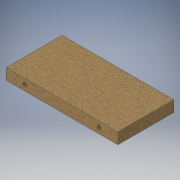
# Autodesk Inventor part: AkkuHaltSeitenWand
Saved by Autodesk Inventor 2017 SP1 (Build 210196100, 196)
## iProperties
Part Number: AkkuHaltSeitenWand
Material: Generisch
Document SubType Name: Modeling
Designer: Alex
Density: 1 g/cm^3
Appearance: Vorgabe
Author: Alex
Autodesk Inventor part; units mm, degrees
ref_plane "YZ Plane" through (0, 0, 0) normal (1, 0, 0) x (0, 1, 0)
ref_plane "XZ Plane" through (0, 0, 0) normal (0, 1, 0) x (-1, 0, 0)
ref_plane "XY Plane" through (0, 0, 0) normal (0, 0, 1) x (1, 0, 0)
sketch "Skizze1" plane through (0, 0, 0) normal (0, 1, 0) x (-1, 0, 0)
  line L0 (0, 0) -> (60, 0)
  line L1 (60, 0) -> (60, -6)
  line L2 (60, -6) -> (0, -6)
  line L3 (0, -6) -> (0, 0)
  dimension "d0" = 60
  dimension "d1" = 6
  constraints: 8 end point, 2 parallel, 1 horizontal, 1 perpendicular
  measures "d0" distance of L1.end L2.end
  measures "d1" distance of L0.end L1.end
extrude "Extrusion1" add sketch "Skizze1" along normal blind 30
sketch "m" plane through (0, 0, 0) normal (0, -1, 0) x (1, 0, 0)
  line L0 (0, -6) -> (0, 0) projected
  line L1 (-60, -6) -> (0, -6) projected
  point P0 (-10, -3)
  point P1 (-50, -3)
  dimension "d4" = 40
  dimension "d5" = 10
  dimension "d6" = 3
  constraints: 1 horizontal alignment
  measures "d4" distance of point (-50, -3) point (-10, -3)
  measures "d5" distance from line of L0 point (-10, -3)
  measures "d6" distance from line of L1 point (-10, -3)
hole "Bohrung1" at (-10, 0, -3) at (-50, 0, -3) direction (0, 1, 0) diameter 2 depth 10 tip angle 118
sketch "Skizze3" plane through (0, 30, 0) normal (0, 1, 0) x (1, 0, 0)
  point P0 (0, 0)
  point P1 (-10, 3)
  point P2 (-50, 3)
hole "Bohrung2" at (-10, 30, -3) at (-50, 30, -3) direction (0, -1, 0) diameter 2 depth 10 tip angle 118
